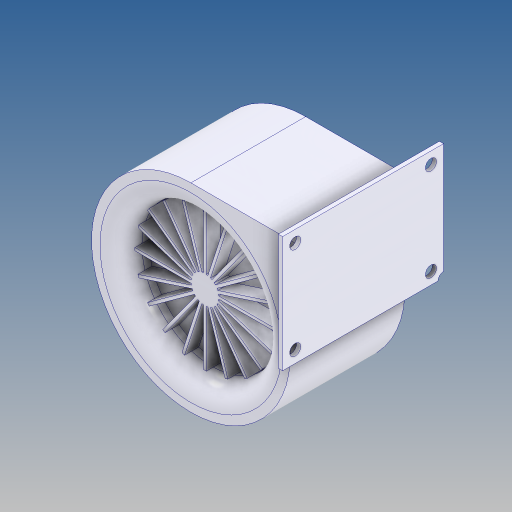
# Autodesk Inventor part: Lüfter G1G108-AB17-02 1,0
Saved by Autodesk Inventor 2023.3 (Build 273359000, 359)
## iProperties
Created: 2024-01-25
Part Number: Lüfter G1G108-AB17-02 1,0
Material: Generisch
Document SubType Name: Modeling
Designer: baerchri
Density: 1 g/cm^3
Appearance: Kühles Weiß
Author: baerchri
Autodesk Inventor part; units mm, degrees
ref_plane "YZ Plane" through (0, 0, 0) normal (1, 0, 0) x (0, 1, 0)
ref_plane "XZ Plane" through (0, 0, 0) normal (0, 1, 0) x (-1, 0, 0)
ref_plane "XY Plane" through (0, 0, 0) normal (0, 0, 1) x (1, 0, 0)
sketch "Skizze1" plane through (0, 0, 0) normal (0, 0, 1) x (1, 0, 0)
  circle A0 centre (0, 0) radius 71
  line L0 (0, 71) -> (79, 71)
  line L1 (79, 71) -> (79, 20)
  line L2 (79, 20) -> (68.1249, 20)
  dimension "d0" = 142
  dimension "d1" = 20
  dimension "d2" = 79
  constraints: 6 end point, 2 perpendicular, 2 point on circle, 1 centre point, 1 coincident, 1 horizontal, 1 tangent
  measures "d0" diameter of A0
  measures "d1" distance from line of point (0, 0) L2
  measures "d2" distance from line of point (0, 0) L1
extrude "Extrusion1" add sketch "Skizze1" along normal blind 82
sketch "Skizze2" plane through (0, 0, 82) normal (0, 0, 1) x (1, 0, 0)
  circle A0 centre (0, 0) radius 50
  dimension "d5" = 100
  constraints: 1 centre point, 1 coincident
  measures "d5" diameter of A0
extrude "Extrusion2" cut sketch "Skizze2" against normal blind 20
fillet "Rundung1" radius 15 1 edges at (-50, 0, 82)
sketch "Skizze3" plane through (79, 20, 0) normal (1, 0, 0) x (0, 0, -1)
  line L0 (0, 0) -> (0, 51) projected
  line L1 (0, 51) -> (-82, 51) projected
  line L2 (-82, 0) -> (-82, 51) projected
  line L3 (0, 0) -> (-82, 0) projected
  line L4 (0, 51) -> (-82, 51) projected
  line L5 (-82, 51) -> (0, 0)
  line L6 (0, 0) -> (0, 51) projected
  line L7 (0, 51) -> (-82, 0)
  line L8 (-98.5, 67) -> (16.5, 67)
  line L9 (16.5, 67) -> (16.5, -16)
  line L10 (16.5, -16) -> (-98.5, -16)
  line L11 (-98.5, -16) -> (-98.5, 67)
  line L12 (-98.5, 67) -> (16.5, -16) construction
  line L13 (16.5, 67) -> (-98.5, -16) construction
  point P0 (0, -20)
  point P1 (-41, 25.5)
  dimension "d9" = 115
  dimension "d10" = 83
  constraints: 16 end point, 3 midpoint, 2 parallel, 1 horizontal, 1 perpendicular
  measures "d9" distance of L9.end L10.end
  measures "d10" distance of L8.end L9.end
extrude "Extrusion3" add sketch "Skizze3" along normal blind 3 contours L5 L7 L0 | L3 L7 L5 | L7 L5 L1 | L2 L5 L7 | L8 L9 L10 L11
sketch "Skizze4" plane through (82, 20, 0) normal (1, 0, 0) x (0, 0, -1)
  line L0 (-98.5, 67) -> (-98.5, -16) projected
  line L1 (-98.5, 67) -> (16.5, -16)
  line L2 (16.5, -16) -> (16.5, 67) projected
  line L3 (16.5, 67) -> (-98.5, -16)
  line L4 (-89.5, -7.5) -> (7.5, -7.5)
  line L5 (7.5, -7.5) -> (7.5, 58.5)
  line L6 (7.5, 58.5) -> (-89.5, 58.5)
  line L7 (-89.5, 58.5) -> (-89.5, -7.5)
  line L8 (-89.5, -7.5) -> (7.5, 58.5) construction
  line L9 (7.5, -7.5) -> (-89.5, 58.5) construction
  point P0 (0, -20)
  point P1 (-41, 25.5)
  dimension "d13" = 97
  dimension "d14" = 66
  constraints: 16 end point, 3 midpoint, 2 parallel, 1 horizontal, 1 perpendicular
  measures "d13" distance of L6.end L5.end
  measures "d14" distance of L5.end L4.end
hole "Bohrung1" at (82, 4, -16.5) at (82, 78.5, 89.5) at (82, 78.5, -7.5) at (82, 12.5, -7.5) at (82, 12.5, 89.5) direction (-1, 0, 0) diameter 8 end through all
sketch "Skizze5" plane through (0, 0, 62) normal (0, 0, 1) x (1, 0, 0)
  line L0 (0, 0) -> (-0.0005, 50)
  circle A0 centre (0, 0) radius 50 projected
  circle A1 centre (0, 0) radius 10
  line L1 (0.9999, 9.9499) -> (0.9995, 49.99)
  line L2 (-1.0001, 9.9499) -> (-1.0005, 49.99)
  dimension "d22" = 20
  dimension "d23" = 2
  dimension "d24" = 1
  constraints: 6 end point, 5 point on circle, 1 centre point, 1 coincident, 1 parallel
  measures "d22" diameter of A1
  measures "d23" distance between parallel lines of L2 L1
  measures "d24" distance between parallel lines of L2 L0
extrude "Extrusion4" add sketch "Skizze5" along normal blind 10 contours A1 L2 A0 L0 | L0 A0 L1 A1 | A1
fillet "Rundung2" radius 5 1 edges at (0.0001, -10, 72)
pattern_circular "Runde Anordnung1" count 20 over 360 about axis through (0, 0, 67) along (0, 0, 1) of "Extrusion4"
equation "\"d24\" = 0.5 * d23"
